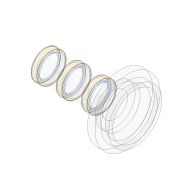
# Autodesk Inventor part: offset_piston
Saved by Autodesk Inventor 2021 (Build 250183000, 183)
## iProperties
Created: 2021-07-12
Part Number: offset_piston
Material: Generic
Document SubType Name: Modeling
Designer: Sihan
Density: 1 g/cm^3
Appearance: Clear Reflective
Mass: 0.924757 g
Surface Area: 14.8287 cm^2
Volume: 0.924757 cm^3
Author: Sihan
Autodesk Inventor part; units mm, degrees
ref_plane "YZ Plane" through (0, 0, 0) normal (1, 0, 0) x (0, 1, 0)
ref_plane "XZ Plane" through (0, 0, 0) normal (0, 1, 0) x (-1, 0, 0)
ref_plane "XY Plane" through (0, 0, 0) normal (0, 0, 1) x (1, 0, 0)
sketch "Sketch1" plane through (0, 0, 0) normal (0, 0, 1) x (1, 0, 0)
  line L0 (-25.6297, 2.5) -> (-25.6297, 2.91)
  line L1 (-25.6297, 2.91) -> (-24.1297, 2.91)
  line L2 (-24.1297, 2.91) -> (-24.1297, 2.5)
  line L3 (-24.1297, 2.5) -> (-20.6297, 2.5)
  line L4 (-20.6297, 2.5) -> (-20.6297, 2.91)
  line L5 (-20.6297, 2.91) -> (-19.1297, 2.91)
  line L6 (-19.1297, 2.91) -> (-19.1297, 2.5)
  line L7 (-19.1297, 2.5) -> (-15.6297, 2.5)
  line L8 (-15.6297, 2.5) -> (-15.6297, 2.91)
  line L9 (-15.6297, 2.91) -> (-14.1297, 2.91)
  line L10 (-14.1297, 2.91) -> (-14.1297, 2.5)
  line L11 (-10.6297, 6.5) -> (-9.1297, 6.5)
  line L12 (-9.1297, 0) -> (-29.6297, 0)
  line L13 (-9.1297, 6.5) -> (-9.1297, 5.3)
  line L14 (-9.1297, 5.3) -> (-7.6297, 5.3)
  line L15 (-7.6297, 5.3) -> (-7.6297, 4.5)
  line L16 (-7.6297, 4.5) -> (-9.1297, 4.5)
  line L17 (-9.1297, 4.5) -> (-9.1297, 0)
  line L18 (-14.1297, 2.5) -> (-11.6297, 2.5)
  line L19 (-11.6297, 2.5) -> (-11.6297, 4)
  line L20 (-11.6297, 4) -> (-10.6297, 4)
  line L21 (-10.6297, 4) -> (-10.6297, 6.5)
  line L22 (-25.6297, 2.5) -> (-25.6297, 0)
  point P0 (0, 0)
  point P1 (-10.1297, 2.5)
  dimension "d2" = 1.5
  dimension "d3" = 1.5
  dimension "d4" = 1.5
  dimension "d5" = 1.5
  dimension "d9" = 3.5
  dimension "d10" = 3.5
  dimension "d14" = 6.5
  dimension "d60" = 5.3
  dimension "d61" = 4.5
  dimension "d62" = 1.5
  dimension "d63" = 2.5
  dimension "d64" = 1
  dimension "d65" = 4
  constraints: 46 end point, 13 perpendicular, 10 point on line, 1 horizontal, 1 vertical
  measures "d2" distance of L0.end L1.end
  measures "d3" distance of L4.end L5.end
  measures "d4" distance of L8.end L9.end
  measures "d5" distance of L11.start L11.end
  measures "d9" distance of L2.end L3.end
  measures "d10" distance of L6.end L7.end
  measures "d14" distance between parallel lines of L12 L11
  measures "d60" distance from line of L12.start L14
  measures "d61" distance from line of L12.start L16
  measures "d62" distance between parallel lines of L17 L15
  measures "d63" distance of L10.end L18.end
  measures "d64" distance of L19.end L20.end
  measures "d65" distance between parallel lines of L12 L20
revolve "Revolution1" add sketch "Sketch1" angle 360 about axis through (-9.1297, 0, 0) along (-1, 0, 0)
sketch "Sketch2" plane through (0, 0, 0) normal (0, 0, 1) x (1, 0, 0)
  line L0 (-34.1297, -2.91) -> (-34.1297, 2.91)
  line L1 (-32.1297, -2.91) -> (-32.1297, 2.91)
  line L2 (-28.1297, -2.91) -> (-28.1297, 2.91)
  line L3 (-26.1297, -2.91) -> (-26.1297, 2.91)
  line L4 (-25.6297, -2.91) -> (-25.6297, 2.91)
  line L5 (-24.1297, -2.91) -> (-24.1297, 2.91)
  line L6 (-20.6297, -2.91) -> (-20.6297, 2.91)
  line L7 (-19.1297, -2.91) -> (-19.1297, 2.91)
  line L8 (-15.6297, -2.91) -> (-15.6297, 2.91)
  line L9 (-14.1297, -2.91) -> (-14.1297, 2.91)
  line L10 (-40.9557, 0) -> (6.8259, 0)
  line L11 (-25.6297, -2.91) -> (-25.6297, 2.91)
  line L12 (-25.6297, 2.91) -> (-24.1297, 2.91)
  line L13 (-24.1297, 2.91) -> (-24.1297, 2.5)
  line L14 (-24.1297, 2.5) -> (-20.6297, 2.5)
  line L15 (-20.6297, 2.5) -> (-20.6297, 2.91)
  line L16 (-19.1297, 2.91) -> (-19.1297, 2.5)
  line L17 (-19.1297, 2.5) -> (-15.6297, 2.5)
  line L18 (-15.6297, 2.5) -> (-15.6297, 2.91)
  line L19 (-14.1297, 2.91) -> (-14.1297, 2.5)
  line L20 (-14.1297, 2.5) -> (-11.6297, 2.5)
  line L21 (-11.6297, 2.5) -> (-11.6297, 4)
  line L22 (-11.6297, 4) -> (-10.6297, 4)
  line L23 (-10.6297, 4) -> (-10.6297, 6.5)
  line L24 (-10.6297, 6.5) -> (-9.1297, 6.5)
  line L25 (-9.1297, 6.5) -> (-9.1297, 5.3)
  line L26 (-9.1297, 5.3) -> (-7.6297, 5.3)
  line L27 (-7.6297, 5.3) -> (-7.6297, 4.5)
  line L28 (-7.6297, 4.5) -> (-9.1297, 4.5)
  line L29 (-9.1297, 4.5) -> (-9.1297, -4.5)
  line L30 (-9.1297, -4.5) -> (-7.6297, -4.5)
  line L31 (-7.6297, -4.5) -> (-7.6297, -5.3)
  line L32 (-7.6297, -5.3) -> (-9.1297, -5.3)
  line L33 (-9.1297, -5.3) -> (-9.1297, -6.5)
  line L34 (-9.1297, -6.5) -> (-10.6297, -6.5)
  line L35 (-10.6297, -6.5) -> (-10.6297, -4)
  line L36 (-10.6297, -4) -> (-11.6297, -4)
  line L37 (-11.6297, -4) -> (-11.6297, -2.5)
  line L38 (-11.6297, -2.5) -> (-14.1297, -2.5)
  line L39 (-14.1297, -2.5) -> (-14.1297, -2.91)
  line L40 (-15.6297, -2.91) -> (-15.6297, -2.5)
  line L41 (-15.6297, -2.5) -> (-19.1297, -2.5)
  line L42 (-19.1297, -2.5) -> (-19.1297, -2.91)
  line L43 (-20.6297, -2.91) -> (-20.6297, -2.5)
  line L44 (-20.6297, -2.5) -> (-24.1297, -2.5)
  line L45 (-24.1297, -2.5) -> (-24.1297, -2.91)
  line L46 (-24.1297, -2.91) -> (-25.6297, -2.91)
  line L47 (-25.6297, -2.91) -> (-25.6297, 2.91)
  line L48 (-25.6297, 2.91) -> (-24.1297, 2.91)
  line L49 (-24.1297, 2.91) -> (-24.1297, 2.5)
  line L50 (-24.1297, 2.5) -> (-20.6297, 2.5)
  line L51 (-14.1297, 2.5) -> (-11.6297, 2.5)
  line L52 (-11.6297, -2.5) -> (-14.1297, -2.5)
  line L53 (-20.6297, -2.5) -> (-24.1297, -2.5)
  line L54 (-24.1297, -2.5) -> (-24.1297, -2.91)
  line L55 (-24.1297, -2.91) -> (-25.6297, -2.91)
  line L56 (-25.6297, 2.91) -> (-24.1297, 2.91)
  arc A0 (-25.3297, 2.91) -> (-24.4297, 2.91) centre (-24.8797, 2.5938) ccw
  line L57 (-20.6297, 2.91) -> (-19.1297, 2.91)
  line L58 (-20.6297, 2.91) -> (-19.1297, 2.91)
  arc A1 (-20.3297, 2.91) -> (-19.4297, 2.91) centre (-19.8797, 2.5938) ccw
  line L59 (-15.6297, 2.91) -> (-14.1297, 2.91)
  line L60 (-15.6297, 2.91) -> (-14.1297, 2.91)
  arc A2 (-15.3297, 2.91) -> (-14.4297, 2.91) centre (-14.8797, 2.5938) ccw
  line L61 (-11.6297, 2.5) -> (-11.6297, 4)
  line L62 (-11.6297, 4) -> (-10.6297, 4)
  line L63 (-10.6297, 4) -> (-10.6297, 6.5)
  line L64 (-10.6297, 6.5) -> (-9.1297, 6.5)
  line L65 (-9.1297, 6.5) -> (-9.1297, 5.3)
  line L66 (-9.1297, 5.3) -> (-7.6297, 5.3)
  line L67 (-7.6297, 5.3) -> (-7.6297, 4.5)
  line L68 (-7.6297, 4.5) -> (-9.1297, 4.5)
  line L69 (-9.1297, 4.5) -> (-9.1297, -4.5)
  line L70 (-9.1297, -4.5) -> (-7.6297, -4.5)
  line L71 (-7.6297, -4.5) -> (-7.6297, -5.3)
  line L72 (-7.6297, -5.3) -> (-9.1297, -5.3)
  line L73 (-9.1297, -5.3) -> (-9.1297, -6.5)
  line L74 (-9.1297, -6.5) -> (-10.6297, -6.5)
  line L75 (-10.6297, -6.5) -> (-10.6297, -4)
  line L76 (-10.6297, -4) -> (-11.6297, -4)
  line L77 (-11.6297, -4) -> (-11.6297, -2.5)
  line L78 (-20.6297, 2.5) -> (-20.6297, 2.91)
  line L79 (-20.6297, 2.91) -> (-19.1297, 2.91)
  line L80 (-19.1297, 2.91) -> (-19.1297, 2.5)
  line L81 (-19.1297, 2.5) -> (-15.6297, 2.5)
  line L82 (-15.6297, 2.5) -> (-15.6297, 2.91)
  line L83 (-15.6297, 2.91) -> (-14.1297, 2.91)
  line L84 (-14.1297, 2.91) -> (-14.1297, 2.5)
  line L85 (-14.1297, -2.5) -> (-14.1297, -2.91)
  line L86 (-14.1297, -2.91) -> (-15.6297, -2.91)
  line L87 (-15.6297, -2.91) -> (-15.6297, -2.5)
  line L88 (-15.6297, -2.5) -> (-19.1297, -2.5)
  line L89 (-19.1297, -2.5) -> (-19.1297, -2.91)
  line L90 (-19.1297, -2.91) -> (-20.6297, -2.91)
  line L91 (-20.6297, -2.91) -> (-20.6297, -2.5)
  line L92 (-20.6297, 2.91) -> (-19.1297, 2.91)
  line L93 (-15.6297, 2.91) -> (-14.1297, 2.91)
  line L94 (-14.1297, -2.91) -> (-15.6297, -2.91)
  line L95 (-19.1297, -2.91) -> (-20.6297, -2.91)
  point P0 (0, 0)
  point P1 (-24.4297, 2.91)
  point P2 (-25.3297, 2.91)
  point P3 (-14.4297, 2.91)
  point P4 (-19.4297, 2.91)
revolve "Revolution2" cut sketch "Sketch2" angle 360 about axis through (-10, 0, 0) along (1, 0, 0) contours L12 A0 | L57 A1 | L59 A2
sketch "Sketch3" plane through (0, 0, 0) normal (0, 0, 1) x (1, 0, 0)
  line L0 (-25.6297, -2.91) -> (-25.6297, 2.91) projected
  line L1 (-25.6297, 2.91) -> (-25.3297, 2.91) projected
  line L2 (-24.1297, 2.91) -> (-24.1297, 2.5) projected
  line L3 (-24.1297, 2.5) -> (-20.6297, 2.5) projected
  line L4 (-20.6297, 2.5) -> (-20.6297, 2.91) projected
  line L5 (-20.6297, 2.91) -> (-20.3297, 2.91) projected
  line L6 (-19.1297, 2.91) -> (-19.1297, 2.5) projected
  line L7 (-19.1297, 2.5) -> (-15.6297, 2.5) projected
  line L8 (-15.6297, 2.5) -> (-15.6297, 2.91) projected
  line L9 (-15.6297, 2.91) -> (-15.3297, 2.91) projected
  line L10 (-14.1297, 2.91) -> (-14.1297, 2.5) projected
  line L11 (-10.6297, 6.5) -> (-9.1297, 6.5) projected
  line L12 (-9.1297, -6.5) -> (-10.6297, -6.5) projected
  line L13 (-14.1297, -2.5) -> (-14.1297, -2.91) projected
  line L14 (-14.1297, -2.91) -> (-14.4297, -2.91) projected
  line L15 (-15.6297, -2.91) -> (-15.6297, -2.5) projected
  line L16 (-15.6297, -2.5) -> (-19.1297, -2.5) projected
  line L17 (-19.1297, -2.5) -> (-19.1297, -2.91) projected
  line L18 (-19.1297, -2.91) -> (-19.4297, -2.91) projected
  line L19 (-20.6297, -2.91) -> (-20.6297, -2.5) projected
  line L20 (-20.6297, -2.5) -> (-24.1297, -2.5) projected
  line L21 (-24.1297, -2.5) -> (-24.1297, -2.91) projected
  line L22 (-24.1297, -2.91) -> (-24.4297, -2.91) projected
  line L23 (-28.7297, 0) -> (-7.0297, 0) projected
  line L24 (-9.1297, 6.5) -> (-9.1297, 5.3) projected
  line L25 (-9.1297, 5.3) -> (-7.6297, 5.3) projected
  line L26 (-7.6297, 5.3) -> (-7.6297, 4.5) projected
  line L27 (-7.6297, 4.5) -> (-9.1297, 4.5) projected
  line L28 (-9.1297, 4.5) -> (-9.1297, -4.5) projected
  line L29 (-9.1297, -4.5) -> (-7.6297, -4.5) projected
  line L30 (-7.6297, -4.5) -> (-7.6297, -5.3) projected
  line L31 (-7.6297, -5.3) -> (-9.1297, -5.3) projected
  line L32 (-9.1297, -5.3) -> (-9.1297, -6.5) projected
  line L33 (-14.1297, 2.5) -> (-11.6297, 2.5) projected
  line L34 (-11.6297, 2.5) -> (-11.6297, 4) projected
  line L35 (-11.6297, 4) -> (-10.6297, 4) projected
  line L36 (-10.6297, 4) -> (-10.6297, 6.5) projected
  line L37 (-10.6297, -6.5) -> (-10.6297, -4) projected
  line L38 (-10.6297, -4) -> (-11.6297, -4) projected
  line L39 (-11.6297, -4) -> (-11.6297, -2.5) projected
  line L40 (-11.6297, -2.5) -> (-14.1297, -2.5) projected
  line L41 (-25.3297, -2.91) -> (-25.6297, -2.91) projected
  arc A0 (-25.3297, 2.91) -> (-24.4297, 2.91) centre (-24.8797, 2.5938) ccw projected
  line L42 (-24.4297, 2.91) -> (-24.1297, 2.91) projected
  arc A1 (-24.6144, 2.2058) -> (-25.145, 2.2058) centre (-24.8797, 2.5938) ccw
  line L43 (-25.0797, 2.082) -> (-25.0797, 2.0814)
  arc A2 (-25.4297, 2.5938) -> (-24.3297, 2.5938) centre (-24.8797, 2.5938) ccw projected
  line L44 (-24.6797, 2.082) -> (-24.6797, 2.0814)
  arc A3 (-25.4297, 2.5938) -> (-24.3297, 2.5938) centre (-24.8797, 2.5938) ccw projected
  arc A4 (-25.0797, 2.082) -> (-25.145, 2.2058) centre (-25.2297, 2.082) ccw
  arc A5 (-24.6144, 2.2058) -> (-24.6797, 2.082) centre (-24.5297, 2.082) ccw
  line L45 (-19.6797, 2.082) -> (-19.6797, 2.0814)
  arc A6 (-19.6144, 2.2058) -> (-19.6797, 2.082) centre (-19.5297, 2.082) ccw
  line L46 (-20.0797, 2.082) -> (-20.0797, 2.0814)
  arc A7 (-20.0797, 2.082) -> (-20.145, 2.2058) centre (-20.2297, 2.082) ccw
  arc A8 (-19.6144, 2.2058) -> (-20.145, 2.2058) centre (-19.8797, 2.5938) ccw
  line L47 (-14.6797, 2.082) -> (-14.6797, 2.0814)
  arc A9 (-14.6144, 2.2058) -> (-14.6797, 2.082) centre (-14.5297, 2.082) ccw
  line L48 (-15.0797, 2.082) -> (-15.0797, 2.0814)
  arc A10 (-15.0797, 2.082) -> (-15.145, 2.2058) centre (-15.2297, 2.082) ccw
  arc A11 (-14.6144, 2.2058) -> (-15.145, 2.2058) centre (-14.8797, 2.5938) ccw
  arc A12 (-24.4297, -2.91) -> (-25.3297, -2.91) centre (-24.8797, -2.5938) ccw projected
  arc A13 (-14.4297, -2.91) -> (-15.3297, -2.91) centre (-14.8797, -2.5938) ccw projected
  line L49 (-15.3297, -2.91) -> (-15.6297, -2.91) projected
  arc A14 (-19.4297, -2.91) -> (-20.3297, -2.91) centre (-19.8797, -2.5938) ccw projected
  line L50 (-20.3297, -2.91) -> (-20.6297, -2.91) projected
  arc A15 (-20.3297, 2.91) -> (-19.4297, 2.91) centre (-19.8797, 2.5938) ccw projected
  line L51 (-19.4297, 2.91) -> (-19.1297, 2.91) projected
  arc A16 (-15.3297, 2.91) -> (-14.4297, 2.91) centre (-14.8797, 2.5938) ccw projected
  line L52 (-14.4297, 2.91) -> (-14.1297, 2.91) projected
  point P0 (-24.4797, 2.91)
  point P1 (-20.4797, 2.91)
  point P2 (-16.4797, 2.91)
  point P3 (-25.0797, 2.1684)
  point P4 (-24.6797, 2.1684)
  point P5 (-19.6797, 2.1684)
  point P6 (-20.0797, 2.1684)
  point P7 (-14.6797, 2.1684)
  point P8 (-15.0797, 2.1684)
  point P9 (-25.0797, 2.0814)
  point P10 (-24.6797, 2.0814)
  point P11 (-24.518, 2.2648)
  point P12 (-25.2414, 2.2648)
  point P13 (-25.0828, 2.1531)
  point P14 (-24.6766, 2.1531)
  dimension "d82" = 0.94
  dimension "d83" = 0.2
  dimension "d84" = 0.2
  dimension "d85" = 0.15
  dimension "d88" = 5
  constraints: 26 point on circle, 12 end point, 9 centre point, 6 point on line, 4 tangent, 1 coincident, 1 equal radius, 1 horizontal, 1 parallel, 1 vertical, 32 other
  measures "d82" diameter of A1
  measures "d83" distance from line of A0.centre L43
  measures "d84" distance from line of A0.centre L44
  measures "d85" radius of A4
  measures "d88" distance of A5.centre A6.centre
revolve "Revolution5" add sketch "Sketch3" angle 360 about axis through (-10, 0, 0) along (1, 0, 0) separate body contours A4 A1 A5 A0 | A7 A8 A6 A15 | A16 A10 A11 A9
chamfer "Chamfer1" distance 0.15 angle 45 3 edges at (-25.6297, -2.91, 0) (-20.6297, -2.91, 0) (-15.6297, -2.91, 0)
chamfer "Chamfer2" distance 0.15 angle 45 3 edges at (-24.1297, -2.91, 0) (-19.1297, -2.91, 0) (-14.1297, -2.91, 0)
fillet "Fillet6" radius 0.05 4 edges at (-25.3297, -2.91, 0) (-24.4297, -2.91, 0) (-19.4297, -2.91, 0) (-14.4297, -2.91, 0)
body "Solid1"
body "Solid4"
